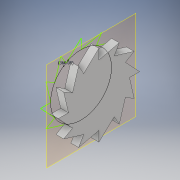
# Autodesk Inventor part: ratchet_gear
Saved by Autodesk Inventor 2017 (Build 210142000, 142)
## iProperties
Created: 2017-01-16
Part Number: ratchet_gear
Material: Generic
Document SubType Name: Modeling
Designer: mmarkle
Density: 1 g/cm^3
Appearance: Default
Author: mmarkle
Autodesk Inventor part; units mm, degrees
ref_plane "XZ Plane" through (0, 0, 0) normal (0, 1, 0) x (-1, 0, 0)
ref_plane "XY Plane" through (0, 0, 0) normal (0, 0, 1) x (1, 0, 0)
sketch "Sketch1" plane through (0, 0, 0) normal (1, 0, 0) x (0, 1, 0)
  line L0 (16.4978, 9.525) -> (25.4, 0)
  line L1 (25.4, 0) -> (19.05, 0)
  line L2 (9.525, 16.4978) -> (21.997, 12.7)
  line L3 (21.997, 12.7) -> (16.4978, 9.525)
  line L4 (0, 19.05) -> (12.7, 21.997)
  line L5 (12.7, 21.997) -> (9.525, 16.4978)
  line L6 (-9.525, 16.4978) -> (0, 25.4)
  line L7 (0, 25.4) -> (0, 19.05)
  line L8 (-16.4978, 9.525) -> (-12.7, 21.997)
  line L9 (-12.7, 21.997) -> (-9.525, 16.4978)
  line L10 (-19.05, 0) -> (-21.997, 12.7)
  line L11 (-21.997, 12.7) -> (-16.4978, 9.525)
  line L12 (-16.4978, -9.525) -> (-25.4, 0)
  line L13 (-25.4, 0) -> (-19.05, 0)
  line L14 (-9.525, -16.4978) -> (-21.997, -12.7)
  line L15 (-21.997, -12.7) -> (-16.4978, -9.525)
  line L16 (0, -19.05) -> (-12.7, -21.997)
  line L17 (-12.7, -21.997) -> (-9.525, -16.4978)
  line L18 (9.525, -16.4978) -> (0, -25.4)
  line L19 (0, -25.4) -> (0, -19.05)
  line L20 (16.4978, -9.525) -> (12.7, -21.997)
  line L21 (12.7, -21.997) -> (9.525, -16.4978)
  line L22 (19.05, 0) -> (21.997, -12.7)
  line L23 (21.997, -12.7) -> (16.4978, -9.525)
  point P0 (0, 0)
  dimension "d7" = 360
  constraints: 48 end point, 1 horizontal, 61 other
ref_plane "Work Plane1" through (6.35, 0, 0) normal (1, 0, 0) x (0, 1, 0)
sketch "Sketch2" plane through (6.35, 0, 0) normal (1, 0, 0) x (0, 1, 0)
  line L0 (21.997, 12.7) -> (16.4978, 9.525)
  line L1 (16.4978, 9.525) -> (25.4, 0)
  line L2 (25.4, 0) -> (19.05, 0)
  line L3 (19.05, 0) -> (21.997, -12.7)
  line L4 (21.997, -12.7) -> (16.4978, -9.525)
  line L5 (16.4978, -9.525) -> (12.7, -21.997)
  line L6 (12.7, -21.997) -> (9.525, -16.4978)
  line L7 (9.525, -16.4978) -> (0, -25.4)
  line L8 (0, -25.4) -> (0, -19.05)
  line L9 (0, -19.05) -> (-12.7, -21.997)
  line L10 (-12.7, -21.997) -> (-9.525, -16.4978)
  line L11 (-9.525, -16.4978) -> (-21.997, -12.7)
  line L12 (-21.997, -12.7) -> (-16.4978, -9.525)
  line L13 (-16.4978, -9.525) -> (-25.4, 0)
  line L14 (-25.4, 0) -> (-19.05, 0)
  line L15 (-19.05, 0) -> (-21.997, 12.7)
  line L16 (-21.997, 12.7) -> (-16.4978, 9.525)
  line L17 (-16.4978, 9.525) -> (-12.7, 21.997)
  line L18 (-12.7, 21.997) -> (-9.525, 16.4978)
  line L19 (-9.525, 16.4978) -> (0, 25.4)
  line L20 (0, 25.4) -> (0, 19.05)
  line L21 (0, 19.05) -> (12.7, 21.997)
  line L22 (12.7, 21.997) -> (9.525, 16.4978)
  line L23 (9.525, 16.4978) -> (21.997, 12.7)
  point P0 (0, 0)
  constraints: 48 end point, 16 perpendicular, 2 collinear, 1 horizontal
extrude "Extrusion1" add sketch "Sketch2" along normal blind 4.826
body "Solid1"
